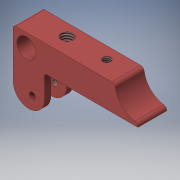
# Autodesk Inventor part: Part2
Saved by Autodesk Inventor 2016 SP1 (Build 200210100, 210)
## iProperties
Created: 2015-12-27
Part Number: Part2
Material: Generic
Document SubType Name: Modeling
Designer: Dirk Alferink
Density: 1 g/cm^3
Appearance: Chestnut
Author: Dirk Alferink
Autodesk Inventor part; units mm, degrees
ref_plane "YZ Plane" through (0, 0, 0) normal (1, 0, 0) x (0, 1, 0)
ref_plane "XZ Plane" through (0, 0, 0) normal (0, 1, 0) x (-1, 0, 0)
ref_plane "XY Plane" through (0, 0, 0) normal (0, 0, 1) x (1, 0, 0)
sketch "Sketch1" plane through (0, 0, 0) normal (0, 1, 0) x (-1, 0, 0)
  line L0 (0, 0) -> (0, 27)
  line L1 (0, 27) -> (-52, 27)
  line L2 (-52, 27) -> (-52, 16)
  line L3 (-52, 16) -> (-13, 16)
  line L4 (-13, 16) -> (-13, 0)
  line L5 (-13, 0) -> (0, 0)
  dimension "d0" = 27
  dimension "d1" = 52
  dimension "d2" = 11
  dimension "d3" = 39
  dimension "d57" = 16
  constraints: 12 end point, 5 perpendicular, 1 vertical
  measures "d0" distance of L0.start L0.end
  measures "d1" distance of L0.end L1.end
  measures "d2" distance of L1.end L2.end
  measures "d3" distance of L2.end L3.end
  measures "d57" distance between parallel lines of L5 L3
extrude "Extrusion1" add sketch "Sketch1" along normal blind 12
sketch "Sketch2" plane through (0, 0, 0) normal (0, -1, 0) x (1, 0, 0)
  line L0 (0, 0) -> (0, 27) projected
  line L1 (0, 27) -> (52, 27) projected
  point P0 (5.5, 21.5)
  dimension "d6" = 5.5
  dimension "d7" = 5.5
  measures "d6" distance from line of L0 point (5.5, 21.5)
  measures "d7" distance from line of L1 point (5.5, 21.5)
hole "Hole1" at (5.5, 0, 21.5) direction (0, 1, 0) diameter 3.5 end through all counterbore diameter 8 counterbore depth 6.5
sketch "Sketch3" plane through (0, 12, 0) normal (0, 1, 0) x (1, 0, 0)
  line L0 (0, 0) -> (0, -27) projected
  line L1 (13, 0) -> (0, 0) projected
  point P0 (8, -5.5)
  dimension "d15" = 8
  dimension "d16" = 5.5
  measures "d15" distance from line of L0 point (8, -5.5)
  measures "d16" distance from line of L1 point (8, -5.5)
hole "Hole2" at (8, 12, 5.5) direction (0, -1, 0) diameter 2.459 end through all thread size "M3x0.5" class "6H" standard "ISO Metric profile"
sketch "Sketch4" plane through (13, 0, 16) normal (1, 0, 0) x (0, 0, -1)
  line L0 (0, 0) -> (0, 12) projected
  line L1 (16, 2.7) -> (0, 2.7)
  line L2 (0, 2.7) -> (0, 9.3)
  line L3 (0, 9.3) -> (16, 9.3)
  line L4 (16, 9.3) -> (16, 2.7)
  line L5 (0, 0) -> (16, 0) projected
  line L6 (0, 12) -> (16, 12) projected
  dimension "d58" = 12
  dimension "d59" = 6.6
  dimension "d60" = 2.7
  constraints: 8 end point, 2 parallel, 1 horizontal, 1 perpendicular, 1 point on line
  measures "d58" distance between parallel lines of L5 L6
  measures "d59" distance of L3.end L1.start
  measures "d60" distance between parallel lines of L3 L6
extrude "Extrusion2" cut sketch "Sketch4" against normal through all
sketch "Sketch5" plane through (0, 0, 27) normal (0, 0, 1) x (1, 0, 0)
  line L0 (0, 0) -> (52, 0) projected
  line L1 (0, 0) -> (0, 12) projected
  point P0 (15.5, 7)
  dimension "d28" = 7
  dimension "d29" = 15.5
  measures "d28" distance from line of L0 point (15.5, 7)
  measures "d29" distance from line of L1 point (15.5, 7)
hole "Hole3" at (15.5, 7, 27) direction (0, 0, -1) diameter 4.917 end through all thread size "M6x1" class "6H" standard "ISO Metric profile"
sketch "Sketch6" plane through (0, 0, 27) normal (0, 0, 1) x (1, 0, 0)
  line L0 (0, 0) -> (52, 0) projected
  line L1 (0, 0) -> (0, 12) projected
  point P0 (32, 7)
  dimension "d37" = 7
  dimension "d38" = 32
  measures "d37" distance from line of L0 point (32, 7)
  measures "d38" distance from line of L1 point (32, 7)
hole "Hole4" at (32, 7, 27) direction (0, 0, -1) diameter 3.242 end through all thread size "M4x0.7" class "6H" standard "ISO Metric profile"
sketch "Sketch7" plane through (0, 0, 0) normal (0, -1, 0) x (1, 0, 0)
  line L0 (0, 27) -> (52, 27) projected
  point P0 (0, 0)
hole "Hole5" at (52, 0, 27) direction (0, 1, 0) diameter 19 end through all
fillet "Fillet1" radius 1.5 2 edges at (42.5, 6, 27) (52, 6, 17.5)
fillet "Fillet2" radius 6.5 4 edges at (13, 1.35, 0) (13, 10.65, 0) (0, 10.65, 0) (0, 1.35, 0)
fillet "Fillet3" radius 1 1 edges at (0, 6, 27)
fillet "Fillet4" radius 1 2 edges at (13, 1.35, 16) (13, 10.65, 16)
equation "\"d60\" = -0.5 * d59 + 0.5 * d58"
body "Solid1"
